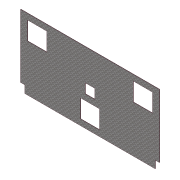
# Autodesk Inventor part: GE-12028-01
Saved by Autodesk Inventor 2012 (Build 160160000, 160)
## iProperties
Created: 2008-05-29
Part Number: GE-12028-01
Description: Panel, Diamond Plate
Document SubType Name: Modeling
Designer: dfoster
Mass: 7964.11 g
Surface Area: 33706.4 cm^2
Volume: 7964.11 cm^3
Density: 1 g/cm^3
Material: Default
Author: narosenberg
Autodesk Inventor part; units mm, degrees
ref_plane "YZ Plane" through (0, 0, 0) normal (1, 0, 0) x (0, 1, 0)
ref_plane "XZ Plane" through (0, 0, 0) normal (0, 1, 0) x (-1, 0, 0)
sketch "Sketch1" plane through (0, 0, 0) normal (0, 0, 1) x (1, 0, 0)
  line L0 (-35.873, 23.0159) -> (1792.927, 23.0159)
  line L1 (1792.927, 23.0159) -> (1792.927, -910.4341)
  line L2 (1792.927, -910.4341) -> (-35.873, -910.4341)
  line L3 (-35.873, -910.4341) -> (-35.873, 23.0159)
  dimension "d0" = 1828.8
  dimension "d1" = 933.45
  constraints: 8 end point, 2 parallel, 1 horizontal, 1 perpendicular
  measures "d0" distance of L0.start L0.end
  measures "d1" distance of L0.end L1.end
extrude "Extrusion1" add sketch "Sketch1" along normal blind 4.7625
ref_plane "Work Plane1" through (0, 0, 6.0325) normal (0, 0, 1) x (1, 0, 0)
sketch "Sketch5" plane through (0, 0, 4.7625) normal (0, 0, 1) x (1, 0, 0)
  line L0 (1792.927, 23.0159) -> (1792.927, -910.4341) projected
  line L1 (-35.873, -910.4341) -> (-35.873, 23.0159) projected
  line L2 (1792.927, -910.4341) -> (-35.873, -910.4341) projected
  line L3 (54.6145, -53.1841) -> (308.6145, -53.1841)
  line L4 (308.6145, -53.1841) -> (308.6145, -294.4841)
  line L5 (308.6145, -294.4841) -> (54.6145, -294.4841)
  line L6 (54.6145, -294.4841) -> (54.6145, -53.1841)
  line L7 (751.527, -592.9341) -> (1005.527, -592.9341)
  line L8 (1005.527, -592.9341) -> (1005.527, -834.2341)
  line L9 (1005.527, -834.2341) -> (751.527, -834.2341)
  line L10 (751.527, -834.2341) -> (751.527, -592.9341)
  line L11 (1448.4395, -53.1841) -> (1702.4395, -53.1841)
  line L12 (1702.4395, -53.1841) -> (1702.4395, -294.4841)
  line L13 (1702.4395, -294.4841) -> (1448.4395, -294.4841)
  line L14 (1448.4395, -294.4841) -> (1448.4395, -53.1841)
  line L15 (-35.873, -910.4341) -> (18.102, -910.4341)
  line L16 (18.102, -910.4341) -> (18.102, -812.0091)
  line L17 (18.102, -812.0091) -> (-35.873, -812.0091)
  line L18 (-35.873, -812.0091) -> (-35.873, -910.4341)
  line L19 (1792.927, -910.4341) -> (1738.952, -910.4341)
  line L20 (1738.952, -910.4341) -> (1738.952, -812.0091)
  line L21 (1738.952, -812.0091) -> (1792.927, -812.0091)
  line L22 (1792.927, -812.0091) -> (1792.927, -910.4341)
  line L23 (815.027, -389.7341) -> (942.027, -389.7341)
  line L24 (942.027, -389.7341) -> (942.027, -516.7341)
  line L25 (942.027, -516.7341) -> (815.027, -516.7341)
  line L26 (815.027, -516.7341) -> (815.027, -389.7341)
  point P0 (0, 0)
  dimension "d55" = 90.4875
  dimension "d56" = 615.95
  dimension "d57" = 76.2
  dimension "d58" = 254
  dimension "d59" = 90.4875
  dimension "d60" = 787.4
  dimension "d61" = 1828.8
  dimension "d64" = 241.3
  dimension "d65" = 254
  dimension "d66" = 241.3
  dimension "d67" = 98.425
  dimension "d68" = 53.975
  dimension "d69" = 127
  dimension "d70" = 63.5
  dimension "d71" = 76.2
  constraints: 48 end point, 12 parallel, 6 horizontal, 6 perpendicular, 4 equal length, 2 collinear
  measures "d55" distance between parallel lines of L6 L1
  measures "d56" distance between parallel lines of L5 L2
  measures "d57" distance between parallel lines of L9 L2
  measures "d58" distance of L4.end L5.end
  measures "d59" distance between parallel lines of L12 L0
  measures "d60" distance between parallel lines of L10 L1
  measures "d61" distance of L0.end L1.start
  measures "d64" distance of L3.end L4.end
  measures "d65" distance of L12.end L13.end
  measures "d66" distance between parallel lines of L11 L13
  measures "d67" distance between parallel lines of L2 L17
  measures "d68" distance between parallel lines of L16 L1
  measures "d69" distance of L23.start L23.end
  measures "d70" distance between parallel lines of L10 L26
  measures "d71" distance between parallel lines of L25 L7
extrude "Extrusion2" cut sketch "Sketch5" against normal blind 25.4
equation "\"d59\" = d55"
equation "\"d60\" = -0.5 * d58 + 0.5 * d61"
equation "\"d65\" = d58"
equation "\"d66\" = d64"
equation "\"d70\" = -0.5 * d69 + 0.5 * d58"
body "Solid1"
